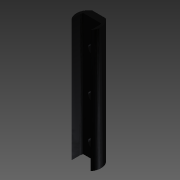
# Autodesk Inventor part: Pasek_reulacji
Saved by Autodesk Inventor 2015 (Build 190159000, 159)
## iProperties
Created: 2015-12-05
Part Number: Pasek_reulacji
Material: Stal nierdzewna
Document SubType Name: Modeling
Designer: graaapsik
Density: 8.08 g/cm^3
Appearance: Gładkie - czarne
Author: graaapsik
Autodesk Inventor part; units mm, degrees
ref_plane "YZ Plane" through (0, 0, 0) normal (1, 0, 0) x (0, 1, 0)
ref_plane "XZ Plane" through (0, 0, 0) normal (0, 1, 0) x (-1, 0, 0)
ref_plane "XY Plane" through (0, 0, 0) normal (0, 0, 1) x (1, 0, 0)
sketch "Szkic1" plane through (0, 0, 0) normal (0, 0, 1) x (1, 0, 0)
  circle A0 centre (0, 0) radius 9
  dimension "d0" = 18
  constraints: 1 centre point, 1 coincident
  measures "d0" diameter of A0
extrude "Wyciągnięcie proste1" add sketch "Szkic1" along normal mid plane 90
sketch "Szkic2" plane through (0, 0, 45) normal (0, 0, 1) x (1, 0, 0)
  circle A0 centre (0, 0) radius 9 projected
  line L0 (-4.9749, 7.5) -> (4.9749, 7.5)
  line L1 (-6.5383, 2.5) -> (6.5383, 2.5)
  line L2 (-6.5, -2.5981) -> (-6.5, -6.2249)
  line L3 (6.5, -2.5981) -> (6.5, -6.2249)
  line L4 (0, 0) -> (0, -2.0526) construction
  arc A1 (-6.5383, 2.5) -> (-6.5, -2.5981) centre (0, 0) ccw
  arc A2 (6.5, -2.5981) -> (6.5383, 2.5) centre (0, 0) ccw
  arc A3 (-6.5, -6.2249) -> (6.5, -6.2249) centre (0, 0) ccw
  arc A4 (4.9749, 7.5) -> (-4.9749, 7.5) centre (0, 0) ccw
  dimension "d3" = 1.5
  dimension "d5" = 5
  dimension "d9" = 2
  dimension "d22" = 13
  constraints: 12 point on circle, 10 end point, 4 centre point, 2 parallel, 1 coincident, 1 horizontal, 1 perpendicular, 1 other
  measures "d3" distance edge to line of A0 L0
  measures "d5" distance between parallel lines of L0 L1
  measures "d9" radial gap between concentric circles of A0 A1
  measures "d22" distance between parallel lines of L3 L2
extrude "Wyciągnięcie proste2" cut sketch "Szkic2" against normal up to next contours L0 A0 | A0 L2 A1 L1 A2 L3
sketch "Szkic3" plane through (-4.9749, 7.5, 45) normal (0, 1, 0) x (1, 0, 0)
  line L0 (9.9499, 0) -> (0, 0) projected
  point P0 (4.9749, 45)
  point P1 (4.9749, 20)
  point P2 (4.9749, 50)
  point P3 (4.9749, 80)
  dimension "d12" = 20
  dimension "d13" = 30
  dimension "d14" = 30
  measures "d12" distance from line of point (4.975, 20) L0
  measures "d13" distance of point (4.975, 50) point (4.975, 20)
  measures "d14" distance of point (4.975, 80) point (4.975, 50)
hole "Otwór1" at (0, 7.5, 25) at (0, 7.5, -5) at (0, 7.5, -35) direction (0, -1, 0) diameter 6 end through all
